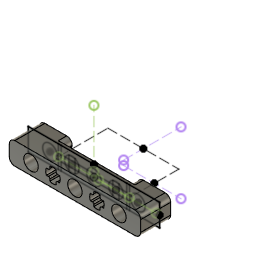
lego (Autodesk Fusion 360 design; units mm, degrees)
Autodesk Fusion 360 part; units mm, degrees
sketch "Sketch1" plane through (0, 0, 0) normal (0, 0, 1) x (1, 0, 0)
  line L0 (-12.825, 8.875) -> (12.825, 8.875) construction
  line L1 (12.825, 8.875) -> (12.825, -8.875) construction
  line L2 (12.825, -8.875) -> (-12.825, -8.875) construction
  line L3 (-12.825, -8.875) -> (-12.825, 8.875) construction
  line L4 (0, 1.75) -> (0, 22.5) construction
  line L5 (1.75, 0) -> (22.5, 0) construction
  point P0 (0, 8.875)
  point P1 (12.825, 0)
  dimension "d1" = 25.65
  dimension "d2" = 17.75
  constraint horizontal L0
  constraint vertical L1
  constraint horizontal L2
  constraint vertical L3
  constraint midpoint L0 P0
  constraint midpoint L1 P1
  constraint coincident P0 L4
  constraint coincident P1 L5
  measures "d1" distance of L0.start L0.end
  measures "d2" distance of L0.start L2.end
ref_plane "WorkPlane1" through (0, -9, 0) normal (0, 1, 0) x (0, 0, 1)
sketch "Sketch2" plane through (0, -9, 0) normal (0, 1, 0) x (1, 0, 0)
  line L0 (-23.75, -4) -> (23.75, -4)
  line L1 (23.75, -4) -> (23.75, 4)
  line L2 (23.75, 4) -> (-23.75, 4)
  line L3 (-23.75, 4) -> (-23.75, -4)
  line L4 (0, -1.75) -> (0, -22.5) construction
  line L5 (1.75, 0) -> (22.5, 0)
  circle A0 centre (0, 0) radius 2.625
  circle A1 centre (7.95, 0) radius 2.625
  circle A2 centre (15.9, 0) radius 2.625
  circle A3 centre (-7.95, 0) radius 2.625
  circle A4 centre (-15.9, 0) radius 2.625
  line L6 (0, 0) -> (7.95, 0) construction
  line L7 (7.95, 0) -> (15.9, 0) construction
  line L8 (-12.875, -4) -> (-12.875, 4)
  line L9 (12.875, -4) -> (12.875, 4)
  line L10 (12.825, 0) -> (-12.825, 0)
  line L11 (-13.5283, 1.125) -> (13.5283, 1.125)
  line L12 (-13.5283, -1.125) -> (13.5283, -1.125)
  line L13 (-6.825, -2.3717) -> (-6.825, 2.3717)
  line L14 (-9.075, -2.3717) -> (-9.075, 2.3717)
  line L15 (-5.5783, -1.125) -> (-5.5783, 1.125) construction
  line L16 (-6.825, -2.3717) -> (-9.075, -2.3717) construction
  line L17 (9.075, -2.3717) -> (9.075, 2.3717)
  line L18 (6.825, -2.3717) -> (6.825, 2.3717)
  line L19 (9.075, -2.3717) -> (6.825, -2.3717) construction
  line L20 (11.875, -4) -> (11.875, 4)
  line L21 (-11.875, -4) -> (-11.875, 4)
  point P0 (0, -4)
  point P1 (23.75, 0)
  dimension "d3" = 47.5
  dimension "d4" = 8
  dimension "d5" = 5.25
  dimension "d6" = 7.95
  dimension "d7" = 25.75
  dimension "d10" = 2.25
  dimension "d24" = 1
  constraint horizontal L0
  constraint vertical L1
  constraint horizontal L2
  constraint vertical L3
  constraint midpoint L0 P0
  constraint midpoint L1 P1
  constraint coincident P0 L4
  constraint coincident P1 L5
  constraint coincident A0.centre L6.start
  constraint coincident L5 A1.centre
  constraint coincident L5 A2.centre
  constraint equal A3 A4
  constraint equal A0 A3
  constraint equal A0 A1
  constraint equal A1 A2
  constraint coincident A1.centre L6.end
  constraint coincident A2.centre L7.end
  constraint parallel L5 L7
  constraint equal L6 L7
  constraint symmetric L4 A1.centre A3.centre
  constraint symmetric L4 A2.centre A4.centre
  constraint coincident L0 L8.start
  constraint coincident L2 L8.end
  constraint perpendicular L2 L8
  constraint coincident L0 L9.start
  constraint coincident L2 L9.end
  constraint perpendicular L2 L9
  constraint symmetric L4 L8.start L9.start
  constraint coincident A4 L11.start
  constraint coincident A2 L11.end
  constraint perpendicular L8 L11
  constraint coincident A4 L12.start
  constraint coincident A2 L12.end
  constraint perpendicular L9 L12
  constraint symmetric L10 L11.end L12.end
  constraint coincident A3 L13.start
  constraint coincident A3 L13.end
  constraint perpendicular L12 L13
  constraint coincident A3 L14.start
  constraint coincident A3 L14.end
  constraint perpendicular L12 L14
  constraint coincident A3 L15.start
  constraint coincident L12 L15.start
  constraint coincident A3 L15.end
  constraint coincident L11 L15.end
  constraint perpendicular L14 L16
  constraint equal L15 L16
  constraint coincident A1 L17.start
  constraint coincident A1 L17.end
  constraint perpendicular L10 L17
  constraint coincident A1 L18.start
  constraint coincident A1 L18.end
  constraint perpendicular L10 L18
  constraint horizontal L19
  constraint equal L16 L19
  constraint coincident L0 L20.start
  constraint coincident L2 L20.end
  constraint perpendicular L2 L20
  constraint coincident L0 L21.start
  constraint coincident L2 L21.end
  constraint perpendicular L2 L21
  constraint symmetric L4 L20.start L21.start
  measures "d3" distance of L0.start L0.end
  measures "d4" distance of L0.end L1.end
  measures "d5" diameter of A0
  measures "d6" distance of A1.centre A0.centre
  measures "d7" distance of L8.end L9.end
  measures "d10" distance of L11 L12
  measures "d24" distance of L9.start L20.start
extrude "Extrude1" add sketch "Sketch2" against normal blind 6.875 contours L0 L2 L3 A4 L8 L11 L12 | L0 L8 L12 L21 | L0 A0 A1 A3 L12 L20 L21 | A4 L8 L11 L12 | L8 L11 L12 L21 | L2 L8 L11 L21 | L0 L9 L12 L20 | A3 L10 L12 L21 | L2 A0 A1 A3 L11 L20 L21 | L0 L1 L2 A2 L9 L11 L12 | L5 L9 L10 L12 L20 | L5 A1 L10 L12 L20 | A3 L12 L14 | A3 L10 L11 L21 | L2 L9 L11 L20 | L5 A2 L9 L12 | A1 L12 L17 | L5 L9 L10 L11 L20 | L5 A1 L10 L11 L20 | A3 L11 L14 | L5 A2 L9 L11 | A3 L12 L13 | A1 L11 L17 | A1 L12 L18 | A0 A3 L10 L12 | A3 L11 L13 | L5 A0 A1 L10 L12 | A0 A3 L10 L11 | A1 L11 L18 | L5 A0 A1 L10 L11
extrude "Extrude2" add sketch "Sketch2" along normal blind 1 contours L0 L2 L3 A4 L8 L11 L12 | L0 L8 L12 L21 | L0 A0 A1 A3 L12 L20 L21 | A4 L8 L11 L12 | L2 L8 L11 L21 | L0 L9 L12 L20 | L2 A0 A1 A3 L11 L20 L21 | L0 L1 L2 A2 L9 L11 L12 | A3 L12 L14 | L2 L9 L11 L20 | L5 A2 L9 L12 | A1 L12 L17 | A3 L11 L14 | L5 A2 L9 L11 | A3 L12 L13 | A1 L11 L17 | A1 L12 L18 | A3 L11 L13 | A1 L11 L18
extrude "Extrude3" add sketch "Sketch2" along normal blind 4 contours L0 L2 L3 A4 L8 L11 L12 | L0 L8 L12 L21 | A4 L8 L11 L12 | L2 L8 L11 L21 | L0 L9 L12 L20 | L0 L1 L2 A2 L9 L11 L12 | L2 L9 L11 L20 | L5 A2 L9 L12 | L5 A2 L9 L11
fillet "Fillet1" radius 2 4 edges at (23.75, -10.4375, 4) (23.75, -10.4375, -4) (-23.75, -10.4375, 4) (-23.75, -10.4375, -4)
fillet "Fillet1" radius 0.5 8 edges at (9.075, -11.9375, 1.125) (6.825, -11.9375, 1.125) (-6.825, -11.9375, 1.125) (-9.075, -11.9375, 1.125) (9.075, -11.9375, -1.125) (6.825, -11.9375, -1.125) (-6.825, -11.9375, -1.125) (-9.075, -11.9375, -1.125)
fillet "Fillet1" radius 2 4 edges at (11.875, -6.5, 4) (11.875, -6.5, -4) (-11.875, -6.5, 4) (-11.875, -6.5, -4)
fillet "Fillet1" radius 0.5 4 edges at (11.875, -6.5, 1.125) (11.875, -6.5, -1.125) (-11.875, -6.5, -1.125) (-11.875, -6.5, 1.125)
equation "d11 = ( -18 / 2 ) * 1 mm"
equation "d12 = ( ( 31.50 - 17.75 ) / 2 ) * -1 mm"
